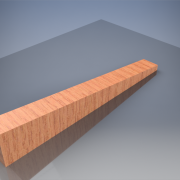
# Autodesk Inventor part: Derby Base
Saved by Autodesk Inventor 2018 (Build 220112000, 112)
## iProperties
Created: 2021-02-22
Part Number: Derby Base
Material: Generic
Document SubType Name: Modeling
Designer: Bell539x
Density: 1 g/cm^3
Appearance: Default
Author: Bell539x
Autodesk Inventor part; units mm, degrees
ref_plane "YZ Plane" through (0, 0, 0) normal (1, 0, 0) x (0, 1, 0)
ref_plane "XZ Plane" through (0, 0, 0) normal (0, 1, 0) x (-1, 0, 0)
ref_plane "XY Plane" through (0, 0, 0) normal (0, 0, 1) x (1, 0, 0)
sketch "Sketch1" plane through (0, 0, 0) normal (1, 0, 0) x (0, 1, 0)
  line L0 (27.097, 129.0528) -> (-4.653, 129.0528)
  line L1 (-4.653, 129.0528) -> (-4.653, -61.4472)
  line L2 (-4.653, -61.4472) -> (1.697, -61.4472)
  line L3 (27.097, 129.0528) -> (1.697, -61.4472)
  point P0 (0, 0)
  dimension "d0" = 31.75
  dimension "d1" = 190.5
  dimension "d2" = 6.35
  constraints: 8 end point, 2 perpendicular, 1 horizontal
  measures "d0" distance of L0.start L0.end
  measures "d1" distance of L0.end L1.end
  measures "d2" distance of L1.end L2.end
extrude "Extrusion1" add sketch "Sketch1" along normal blind 19.05
body "Solid1"
